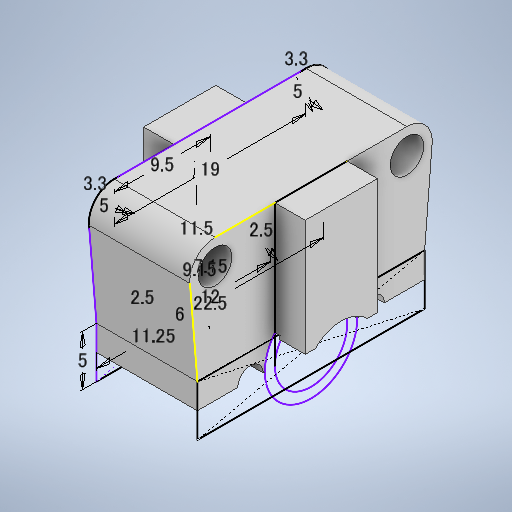
# Autodesk Inventor part: ikafly3c
Saved by Autodesk Inventor 2025 (Build 290162000, 162)
## iProperties
Created: 2024-06-20
Part Number: ikafly3c
Material: 一般
Document SubType Name: Modeling
Designer: Saigusa
Density: 1 g/cm^3
Appearance: 既定
Author: Saigusa
Autodesk Inventor part; units mm, degrees
ref_plane "YZ Plane" through (0, 0, 0) normal (1, 0, 0) x (0, 1, 0)
ref_plane "XZ Plane" through (0, 0, 0) normal (0, 1, 0) x (-1, 0, 0)
ref_plane "XY Plane" through (0, 0, 0) normal (0, 0, 1) x (1, 0, 0)
sketch "スケッチ1" plane through (0, 0, 0) normal (1, 0, 0) x (0, 1, 0)
  circle A0 centre (0, 0) radius 4.575
  circle A1 centre (0, 0) radius 3.575
  line L0 (0, 0) -> (0, 6)
  line L1 (0, 6) -> (0, -6)
  circle A2 centre (0, 6) radius 1.25
  circle A3 centre (0, -6) radius 1.25
  line L2 (0, 0) -> (11.5, 0)
  line L3 (11.5, 0) -> (11.5, 9.5)
  line L4 (11.5, 9.5) -> (11.5, -9.5)
  circle A4 centre (11.5, 9.5) radius 1.65
  circle A5 centre (11.5, -9.5) radius 1.65
  line L5 (0, 0) -> (0, 11.25)
  line L6 (0, 11.25) -> (0, -11.25)
  line L7 (-2.5, -11.25) -> (2.5, -11.25)
  line L8 (2.5, -11.25) -> (2.5, 11.25)
  line L9 (2.5, 11.25) -> (-2.5, 11.25)
  line L10 (-2.5, 11.25) -> (-2.5, -11.25)
  line L11 (-2.5, -11.25) -> (2.5, 11.25) construction
  line L12 (2.5, -11.25) -> (-2.5, 11.25) construction
  circle A6 centre (11.5, 9.5) radius 2.5
  circle A7 centre (11.5, -9.5) radius 2.5
  line L13 (2.5, 11.25) -> (11.2899, 11.9912)
  line L14 (2.5, -11.25) -> (11.2899, -11.9912)
  line L15 (14, 9.5) -> (14, -9.5)
  line L16 (0, -3.575) -> (14, -3.575)
  line L17 (0, 3.575) -> (14, 3.575)
  point P0 (0, 7.25)
  point P1 (0, 4.75)
  point P2 (0, 4.575)
  point P3 (0, -4.575)
  point P4 (0, -4.75)
  point P5 (0, -7.25)
  point P6 (2.5, 3.575)
  point P7 (2.5, 2.5555)
  point P8 (2.5, -2.5555)
  point P9 (2.5, -3.575)
  dimension "d0" = 9.15
  dimension "d1" = 7.15
  dimension "d2" = 6
  dimension "d3" = 12
  dimension "d4" = 2.5
  dimension "d5" = 2.5
  dimension "d6" = 11.5
  dimension "d7" = 9.5
  dimension "d8" = 19
  dimension "d9" = 3.3
  dimension "d10" = 3.3
  dimension "d11" = 11.25
  dimension "d12" = 22.5
  dimension "d13" = 5
  dimension "d14" = 5
  dimension "d15" = 5
  constraints: 36 end point, 8 centre point, 8 coincident, 6 point on circle, 6 point on line, 5 tangent, 4 perpendicular, 2 horizontal, 2 midpoint, 2 parallel, 1 vertical
  measures "d0" diameter of A0
  measures "d1" diameter of A1
  measures "d2" distance of L0.start L0.end
  measures "d3" distance of L0.end L1.end
  measures "d4" diameter of A2
  measures "d5" diameter of A3
  measures "d6" distance of L0.start L2.end
  measures "d7" distance of L2.end L3.end
  measures "d8" distance of L3.end L4.end
  measures "d9" diameter of A4
  measures "d10" diameter of A5
  measures "d11" distance of L0.start L5.end
  measures "d12" distance of L5.end L6.end
  measures "d13" distance of L9.end L8.end
  measures "d14" diameter of A6
  measures "d15" diameter of A7
extrude "押し出し1" add sketch "スケッチ1" along normal blind 10 contours L2 L4 L16 A0 | A0 L17 L3 L2 | A0 L8 L13 A6 L3 L17 | L16 L4 A7 L14 L8 A0 | L3 L17 L15 L16 L4 | A0 L0 A2 L5 L9 L8 | L3 A6 L15 L17 | L8 L7 L6 A3 L1 A0 | L16 L15 A7 L4 | A6 | A7
extrude "押し出し2" add sketch "スケッチ1" against normal blind 3 contours L2 A1 L8 L17 A0 | L2 L4 L16 A0 | A0 L16 L8 A1 L2 | A0 L17 L3 L2 | L3 L17 L15 L16 L4
sketch "スケッチ2" plane through (10, 0, 0) normal (1, 0, 0) x (0, 0, -1)
  circle A0 centre (0, 0) radius 3.575
  line L0 (-3.575, 14) -> (-9.5, 14) projected
  line L1 (-3.575, 0) -> (-3.575, 14)
  line L2 (3.575, 2.8548) -> (3.575, 14) projected
  line L3 (-3.575, 14) -> (3.575, 14)
  line L4 (3.575, 14) -> (3.575, 0)
  line L5 (-11.9912, 11.2899) -> (-11.25, 2.5) projected
  line L6 (11.25, -2.5) -> (-11.25, -2.5)
  line L7 (-11.25, -2.5) -> (-11.25, 2.5)
  line L8 (-11.25, 2.5) -> (11.25, 2.5)
  line L9 (11.25, 2.5) -> (11.25, -2.5)
  line L10 (11.25, -2.5) -> (-11.25, 2.5) construction
  line L11 (-11.25, -2.5) -> (11.25, 2.5) construction
  circle A1 centre (0, 0) radius 4.575
  point P0 (-3.575, 2.8548)
  point P1 (-3.575, 2.5)
  point P2 (-2.5555, 2.5)
  point P3 (2.5555, 2.5)
  point P4 (3.575, 2.5)
  constraints: 18 end point, 3 perpendicular, 2 centre point, 2 coincident, 2 midpoint, 2 parallel, 2 point on circle, 1 horizontal, 1 tangent
extrude "押し出し4" add sketch "スケッチ2" along normal blind 0.5 contours A1 L1 L3 L2
extrude "押し出し5" add sketch "スケッチ2" along normal blind 3 contours A0 L8 L1 A1 L4 | A1 L1 L3 L2
extrude "押し出し6" cut sketch "スケッチ2" along normal blind 0.5 contours A0 L8 L1 A1 L4
